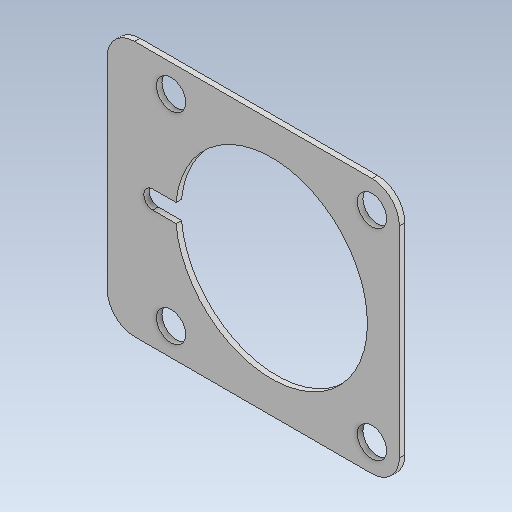
# Autodesk Inventor part: Peça34
Saved by Autodesk Inventor 2021 (Build 250183000, 183)
## iProperties
Category: 41
Created: 2021-07-27
Part Number: Peça34
Material: Genérico
Document SubType Name: Modeling
Designer: Giovanni
Density: 1 g/cm^3
Appearance: Padrão
User Status: 1:2
Author: Giovanni
Keywords: 11
Autodesk Inventor part; units mm, degrees
ref_plane "YZ Plane" through (0, 0, 0) normal (1, 0, 0) x (0, 1, 0)
ref_plane "XZ Plane" through (0, 0, 0) normal (0, 1, 0) x (-1, 0, 0)
ref_plane "XY Plane" through (0, 0, 0) normal (0, 0, 1) x (1, 0, 0)
sketch "Esboço1" plane through (0, 0, 0) normal (0, 0, 1) x (1, 0, 0)
  line L0 (-90, -70) -> (70, -70)
  line L1 (70, -70) -> (70, 70)
  line L2 (70, 70) -> (-90, 70)
  line L3 (-90, 70) -> (-90, -70)
  circle A0 centre (0, 0) radius 52.5
  point P0 (70, 0)
  dimension "d0" = 140
  dimension "d1" = 160
  dimension "d2" = 70
  dimension "d3" = 105
  constraints: 8 end point, 2 parallel, 1 centre point, 1 coincident, 1 horizontal, 1 horizontal alignment, 1 midpoint, 1 perpendicular
  measures "d0" distance of L0.end L1.end
  measures "d1" distance of L0.start L0.end
  measures "d2" distance from line of L1 point (0, 0)
  measures "d3" diameter of A0
extrude "Extrusão1" add sketch "Esboço1" along normal blind 3
sketch "Esboço2" plane through (0, 0, 3) normal (0, 0, 1) x (1, 0, 0)
  line L0 (70, -70) -> (70, 70) projected
  line L1 (70, 70) -> (-90, 70) projected
  line L2 (-90, -70) -> (70, -70) projected
  circle A0 centre (-55, 55) radius 8
  circle A1 centre (55, 55) radius 8
  circle A2 centre (55, -55) radius 8
  circle A3 centre (-55, -55) radius 8
  dimension "d6" = 16
  dimension "d7" = 15
  dimension "d8" = 15
  dimension "d9" = 15
  dimension "d10" = 15
  dimension "d11" = 110
  constraints: 4 centre point, 3 equal radius, 2 horizontal alignment, 2 vertical alignment
  measures "d6" diameter of A1
  measures "d7" distance from line of A1.centre L0
  measures "d8" distance from line of L1 A1.centre
  measures "d9" distance from line of L0 A2.centre
  measures "d10" distance from line of L2 A2.centre
  measures "d11" distance of A0.centre A1.centre
extrude "Extrusão2" cut sketch "Esboço2" against normal up to next
sketch "Esboço3" plane through (0, 0, 3) normal (0, 0, 1) x (1, 0, 0)
  circle A0 centre (0, 0) radius 52.5 projected
  arc A1 (-65, 5) -> (-65, -5) centre (-65, 0) ccw
  line L0 (-65, 5) -> (-45, 5)
  line L1 (-45, 5) -> (-45, -5)
  line L2 (-45, -5) -> (-65, -5)
  dimension "d14" = 65
  dimension "d15" = 5
  dimension "d16" = 20
  constraints: 6 end point, 2 point on circle, 2 tangent, 1 centre point, 1 horizontal, 1 horizontal alignment
  measures "d14" distance of A0.centre A1.centre
  measures "d15" radius of A1
  measures "d16" distance from line of L1 A1.centre
extrude "Extrusão3" cut sketch "Esboço3" against normal up to next contours L0 L1 L2 A0 | A0 L2 A1 L0 picked at (-47.4912, 0.5563)
fillet "Arredondamento1" radius 15 4 edges at (70, 70, 1.5) (70, -70, 1.5) (-90, -70, 1.5) (-90, 70, 1.5)
